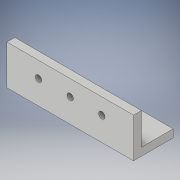
# Autodesk Inventor part: jigproto1 2018ver
Saved by Autodesk Inventor 2018 (Build 220112000, 112)
## iProperties
Created: 2018-12-05
Part Number: jigproto1 2018ver
Material: Generic
Document SubType Name: Modeling
Designer: s-2513225
Density: 1 g/cm^3
Appearance: Default
Author: s-2513225
Autodesk Inventor part; units mm, degrees
ref_plane "YZ Plane" through (0, 0, 0) normal (1, 0, 0) x (0, 1, 0)
ref_plane "XZ Plane" through (0, 0, 0) normal (0, 1, 0) x (-1, 0, 0)
ref_plane "XY Plane" through (0, 0, 0) normal (0, 0, 1) x (1, 0, 0)
sketch "Sketch1" plane through (0, 0, 0) normal (0, 0, 1) x (1, 0, 0)
  line L0 (0, 0) -> (101.6, 0)
  line L1 (101.6, 0) -> (101.6, 25.4)
  line L2 (101.6, 25.4) -> (0, 25.4)
  line L3 (0, 25.4) -> (0, 0)
  line L4 (0, 12.7) -> (101.6, 12.7) construction
  line L5 (50.8, 25.4) -> (50.8, 0) construction
  line L6 (101.6, 24.1606) -> (76.2, 24.1606) construction
  line L7 (76.2, 24.1606) -> (50.8, 24.1606) construction
  line L8 (50.8, 24.1606) -> (25.4, 24.1606) construction
  line L9 (25.4, 24.1606) -> (0, 24.1606) construction
  circle A0 centre (25.4, 12.7) radius 2.5797
  circle A1 centre (50.8, 12.7) radius 2.5797
  circle A2 centre (76.2, 12.7) radius 2.5797
  dimension "d0" = 101.6
  dimension "d1" = 25.4
  dimension "d2" = 25.4
  dimension "d3" = 25.4
  dimension "d4" = 25.4
  dimension "d5" = 5.1594
  dimension "d6" = 5.1594
  dimension "d7" = 5.1594
  constraints: 20 end point, 7 point on line, 5 midpoint, 3 centre point, 2 parallel, 2 perpendicular, 1 horizontal
  measures "d0" distance of L2.end L1.end
  measures "d1" distance of L1.end L0.end
  measures "d2" distance of L6.start L6.end
  measures "d3" distance of L6.end L7.end
  measures "d4" distance of L7.end L8.end
  measures "d5" diameter of A0
  measures "d6" diameter of A1
  measures "d7" diameter of A2
extrude "Extrusion1" add sketch "Sketch1" along normal blind 6.35
sketch "Sketch2" plane through (0, 0, 6.35) normal (0, 0, 1) x (1, 0, 0)
  line L0 (0, 0) -> (101.6, 0) projected
  line L1 (0, 0) -> (101.6, 0)
  line L2 (101.6, 0) -> (101.6, -6.35)
  line L3 (101.6, -6.35) -> (0, -6.35)
  line L4 (0, -6.35) -> (0, 0)
  dimension "d10" = 6.35
  dimension "d11" = 101.6
  constraints: 8 end point, 2 parallel, 1 horizontal, 1 perpendicular
  measures "d10" distance of L1.end L2.end
  measures "d11" distance of L2.end L3.end
extrude "Extrusion2" add sketch "Sketch2" against normal blind 31.75
body "Solid1"
